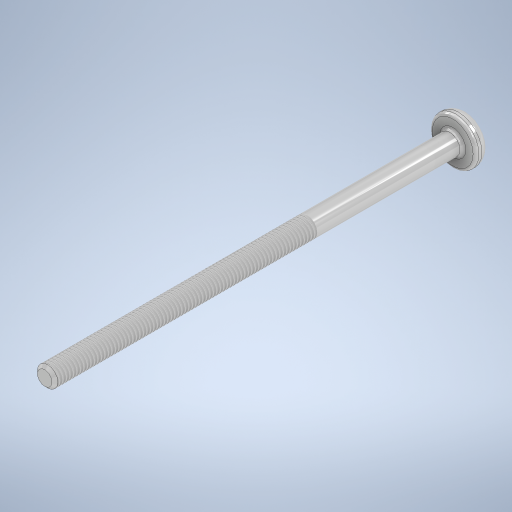
# Autodesk Inventor part: screw
Saved by Autodesk Inventor 2023.2 (Build 272271000, 271)
## iProperties
Created: 2022-11-27
Part Number: screw
Material: Generic
Document SubType Name: Modeling
Designer: omrfrkmll
Density: 1 g/cm^3
Appearance: Aluminum - Dark
Author: omrfrkmll
Autodesk Inventor part; units mm, degrees
ref_plane "YZ Plane" through (0, 0, 0) normal (1, 0, 0) x (0, 1, 0)
ref_plane "XZ Plane" through (0, 0, 0) normal (0, 1, 0) x (-1, 0, 0)
ref_plane "XY Plane" through (0, 0, 0) normal (0, 0, 1) x (1, 0, 0)
sketch "Sketch1" plane through (0, 0, 0) normal (0, 0, 1) x (1, 0, 0)
  circle A0 centre (0, 0) radius 4
  dimension "d0" = 8
  constraints: 1 centre point, 1 coincident
  measures "d0" diameter of A0
extrude "Extrusion1" add sketch "Sketch1" along normal blind 2.5
sketch "Sketch2" plane through (0, 0, 2.5) normal (0, 0, 1) x (1, 0, 0)
  circle A0 centre (0, 0) radius 1.75
  dimension "d3" = 3.5
  constraints: 1 centre point, 1 coincident
  measures "d3" diameter of A0
extrude "Extrusion2" add sketch "Sketch2" along normal blind 70
thread "Thread1" size "M3.5x0.6" class "6g" standard "ANSI Metric M Profile" length 45 offset 25
chamfer "Chamfer1" distance 0.5 angle 45 1 edges at (-1.75, 0, 72.5)
fillet "Fillet1" radius 0.5 1 edges at (-1.75, 0, 2.5)
fillet "Fillet2" radius 1.5 1 edges at (-4, 0, 0)
sketch "Sketch3" plane through (0, 0, 0) normal (0, 0, -1) x (-1, 0, 0)
  line L0 (-1.9955, 1.419) -> (0.9534, 1.419) construction
  line L1 (0.9534, 1.419) -> (0.9534, -1.1751) construction
  line L2 (0.9534, -1.1751) -> (-1.9955, -1.1751) construction
  line L3 (-1.9955, -1.1751) -> (-1.9955, 1.419) construction
  line L4 (1.5864, -0.3671) -> (0.2314, -0.3671)
  line L5 (0.2314, -0.3671) -> (0.2314, -1.722)
  line L6 (0.2314, -1.722) -> (-0.2159, -1.722)
  line L7 (-0.2159, -1.722) -> (-0.2159, -0.3671)
  line L8 (-0.2159, -0.3671) -> (-1.5708, -0.3671)
  line L9 (-1.5708, -0.3671) -> (-1.5708, 0.064)
  line L10 (-1.5708, 0.064) -> (-0.2159, 0.064)
  line L11 (-0.2159, 0.064) -> (-0.2159, 1.419)
  line L12 (-0.2159, 1.419) -> (0.2314, 1.419)
  line L13 (0.2314, 1.419) -> (0.2314, 0.064)
  line L14 (0.2314, 0.064) -> (1.5864, 0.064)
  line L15 (1.5864, 0.064) -> (1.5864, -0.3671)
  point P0 (0, 0)
  constraints: 2 other
emboss "Emboss1" sketch "Sketch3" operation cut depth 2 direction (0, 0, 1)
chamfer "Chamfer2" distance 0.5 angle 45 12 edges at (-0.2314, 0.7415, 0) (-0.9089, 0.064, 0) (-0.9089, -0.3671, 0) (-0.2314, -1.0445, 0) (0.2159, -1.0445, 0) (0.8934, -0.3671, 0) (0.8934, 0.064, 0) (0.2159, 0.7415, 0) (-0.0078, 1.419, 0) (-1.5864, -0.1515, 0) (-0.0078, -1.722, 0) (1.5708, -0.1515, 0)
fillet "Fillet3" radius 0.5 1 edges at (-4, 0, 2.5)
body "Solid1"
